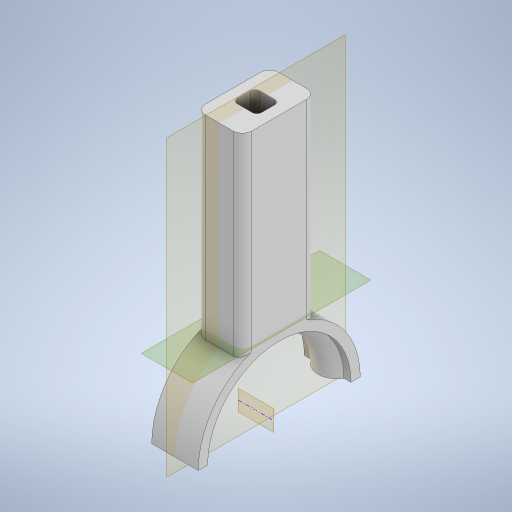
# Autodesk Inventor part: 막대3
Saved by Autodesk Inventor 2023 (Build 270158000, 158)
## iProperties
Created: 2023-04-26
Part Number: 막대3
Material: 일반
Document SubType Name: Modeling
Designer: rlatk
Density: 1 g/cm^3
Appearance: 기본값
Author: rlatk
Autodesk Inventor part; units mm, degrees
ref_plane "XZ Plane" through (0, 0, 0) normal (0, 1, 0) x (-1, 0, 0)
ref_plane "작업 평면1" through (0, 0, 11.4) normal (0, 0, 1) x (1, 0, 0)
sketch "스케치2" plane through (0, 0, 11.4) normal (0, 0, 1) x (1, 0, 0)
  line L0 (-3.8254, 0) -> (3.8254, 0)
  point P0 (0, 0)
  constraints: 2 end point, 1 horizontal
sketch "스케치1" plane through (0, 0, 0) normal (0, 1, 0) x (-1, 0, 0)
  line L0 (0, -4) -> (3.5, -4)
  line L1 (3.5, -4) -> (-3.5, -4)
  arc A0 (3.5, -4) -> (-3.5, -4) centre (0, -5.9365) ccw
  line L2 (0, -9.48) -> (0, 14.88) projected
  line L3 (0, -4) -> (0, -6)
  line L4 (0, -6) -> (5, -6)
  line L5 (5, -6) -> (5, -4)
  line L6 (5, -4) -> (3.5, -4)
  line L7 (0, -4) -> (-5, -4)
  line L8 (-5, -4) -> (-5, -6)
  line L9 (-5, -6) -> (0, -6)
  point P0 (0, -1.9365)
  point P1 (-3.5, -4)
  dimension "d0" = 3.5
  dimension "d1" = 3.5
  dimension "d2" = 4
  dimension "d60" = 2
  dimension "d61" = 5
  dimension "d62" = 2
  dimension "d63" = 5
  dimension "d64" = 2
  constraints: 18 end point, 3 perpendicular, 3 point on circle, 2 point on line, 1 centre point, 1 collinear, 1 midpoint, 1 parallel
  measures "d0" distance of L0.start L0.end
  measures "d1" distance of L0.start L1.end
  measures "d2" radius of A0
  measures "d60" distance of L3.start L3.end
  measures "d61" distance of L3.end L4.end
  measures "d62" distance of L4.end L5.end
  measures "d63" distance of L3.start L7.end
  measures "d64" distance of L7.end L8.end
revolve "회전1" add sketch "스케치1" angle 180 about axis through (-3.8254, 0, 11.4) along (1, 0, 0)
ref_plane "작업 평면3" through (0, 17.4, 11.4) normal (0, -1, 0) x (1, 0, 0)
sketch "스케치12" plane through (0, 17.4, 11.4) normal (0, -1, 0) x (1, 0, 0)
  line L0 (-5, -17.4) -> (-5, 17.4) projected
  line L1 (5, -15.4) -> (5, 15.4) projected
  line L2 (-5, 7.9) -> (5, 7.9)
  line L3 (5, 7.9) -> (5, -7.9)
  line L4 (5, -7.9) -> (-5, -7.9)
  line L5 (-5, -7.9) -> (-5, 7.9)
  line L6 (-7, 0) -> (7, 0) projected
  point P0 (0, -11.4)
  point P1 (5, 7.9)
  point P2 (-5, -7.9)
  dimension "d65" = 7.9
  dimension "d66" = 7.9
  constraints: 8 end point, 2 parallel, 2 point on line, 1 horizontal, 1 perpendicular
  measures "d65" distance between parallel lines of L6 L2
  measures "d66" distance between parallel lines of L4 L6
extrude "돌출12" add sketch "스케치12" against normal blind 40
sketch "스케치13" plane through (0, 0, 0) normal (1, 0, 0) x (0, 1, 0)
  line L0 (17.4, 11.4) -> (17.4, 19.3) projected
  line L1 (17.4, 19.3) -> (57.4, 19.3) projected
  line L2 (17.4, 19.3) -> (17.4, 12.0814)
  line L3 (17.4, 3.5) -> (17.4, 11.4) projected
  line L4 (17.4, 12.0814) -> (17.4, 3.5)
  line L5 (17.4, 3.5) -> (15.5032, 3.5)
  arc A0 (0, -6) -> (17.4, 11.4) centre (0, 11.4) ccw projected
  arc A1 (17.4, 11.4) -> (0, 28.8) centre (0, 11.4) ccw projected
  arc A2 (15.5032, 3.5) -> (17.4, 11.4) centre (0, 11.4) ccw
  line L6 (17.4, 19.3) -> (15.5032, 19.3)
  line L7 (17.4, 19.3) -> (17.4, 11.4)
  arc A3 (17.4, 11.4) -> (15.5032, 19.3) centre (0, 11.4) ccw
  point P0 (0, 0)
  constraints: 10 end point, 6 point on circle, 2 centre point, 2 collinear, 2 concentric, 2 perpendicular, 1 point on line, 1 tangent, 1 vertical
extrude "돌출13" add sketch "스케치13" along normal blind 5 and the other way blind 5
sketch "스케치14" plane through (0, 57.4, 11.4) normal (0, 1, 0) x (1, 0, 0)
  line L0 (5, -7.9) -> (-5, -7.9) projected
  line L1 (-5, 7.9) -> (5, 7.9) projected
  line L2 (3, -7.9) -> (-3, -7.9)
  line L3 (-5, -5.9) -> (-5, 5.9)
  line L4 (-3, 7.9) -> (3, 7.9)
  line L5 (5, 5.9) -> (5, -5.9)
  line L6 (-2.6, -1.4) -> (-2.6, 1.4)
  line L7 (2.6, 1.4) -> (2.6, -1.4)
  line L8 (1.6, -2.4) -> (-1.6, -2.4)
  line L9 (1.6, 2.4) -> (-1.6, 2.4)
  line L10 (7, 0) -> (-7, 0) projected
  arc A0 (3, -7.9) -> (5, -5.9) centre (3, -5.9) ccw
  arc A1 (5, 5.9) -> (3, 7.9) centre (3, 5.9) ccw
  arc A2 (-3, 7.9) -> (-5, 5.9) centre (-3, 5.9) ccw
  arc A3 (-5, -5.9) -> (-3, -7.9) centre (-3, -5.9) ccw
  arc A4 (1.6, -2.4) -> (2.6, -1.4) centre (1.6, -1.4) ccw
  arc A5 (2.6, 1.4) -> (1.6, 2.4) centre (1.6, 1.4) ccw
  arc A6 (-1.6, 2.4) -> (-2.6, 1.4) centre (-1.6, 1.4) ccw
  arc A7 (-2.6, -1.4) -> (-1.6, -2.4) centre (-1.6, -1.4) ccw
  point P0 (0, 11.4)
  point P1 (-2.6, -2.4)
  point P2 (2.6, 2.4)
  point P3 (2.6, -2.4)
  point P4 (-2.6, 2.4)
  dimension "d73" = 2.4
  dimension "d74" = 2.4
  dimension "d75" = 2.4
  dimension "d78" = 2
  dimension "d79" = 1
  dimension "d80" = 1
  dimension "d81" = 1
  dimension "d82" = 1
  dimension "d84" = 5.2
  constraints: 16 end point, 16 point on circle, 16 tangent, 12 point on line, 8 centre point, 4 parallel, 3 equal radius, 2 perpendicular, 1 horizontal
  measures "d73" distance between parallel lines of L5 L7
  measures "d74" distance between parallel lines of L9 L10
  measures "d75" distance between parallel lines of L10 L8
  measures "d78" radius of A0
  measures "d79" radius of A4
  measures "d80" radius of A5
  measures "d81" radius of A6
  measures "d82" radius of A7
  measures "d84" distance between parallel lines of L7 L6
extrude "돌출14" cut sketch "스케치14" against normal blind 50 contours L10 L6 A6 L9 A5 L7 | L7 A4 L8 A7 L6 L10
fillet "모깎기3" radius 2 4 edges at (5, 36.4516, 19.3) (5, 36.4516, 3.5) (-5, 36.4516, 3.5) (-5, 36.4516, 19.3)
sketch "스케치15" plane through (-5, 0, -6) normal (-1, 0, 0) x (0, 0, 1)
  line L0 (19.8, 57.4) -> (19.8, 13.4581) projected
  line L1 (15, 57.4) -> (15, 13.4581) projected
  line L2 (18.8, 18.1404) -> (16, 18.1404)
  line L3 (15, 19.1404) -> (15, 19.5404)
  line L4 (16, 20.5404) -> (18.8, 20.5404)
  line L5 (19.8, 19.5404) -> (19.8, 19.1404)
  arc A0 (18.8, 18.1404) -> (19.8, 19.1404) centre (18.8, 19.1404) ccw
  arc A1 (19.8, 19.5404) -> (18.8, 20.5404) centre (18.8, 19.5404) ccw
  arc A2 (16, 20.5404) -> (15, 19.5404) centre (16, 19.5404) ccw
  arc A3 (15, 19.1404) -> (16, 18.1404) centre (16, 19.1404) ccw
  point P0 (6, 0)
  point P1 (19.8, 18.1404)
  point P2 (15, 20.5404)
  point P3 (17.4, 20.5404)
  point P4 (17.4, 18.1404)
  dimension "d85" = 2.4
  dimension "d86" = 1
  constraints: 8 end point, 8 point on circle, 8 tangent, 6 point on line, 4 centre point, 3 equal radius, 2 midpoint, 2 parallel, 1 horizontal, 1 perpendicular
  measures "d85" distance of point (17.4, 20.54) point (17.4, 18.14)
  measures "d86" radius of A0
extrude "돌출15" cut sketch "스케치15" against normal blind 8
